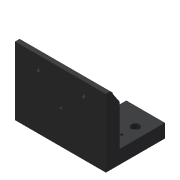
# Autodesk Inventor part: bracket
Saved by Autodesk Inventor 2022 Beta2 (Build 260130000, 130) ContinuousBuild 0
## iProperties
Created: 2006-01-27
Part Number: bracket
Document SubType Name: Modeling
Designer: Dominic
Density: 1 g/cm^3
Material: Generic
Appearance: Generic
Author: dchu
Autodesk Inventor part; units mm, degrees
ref_plane "YZ Plane" through (0, 0, 0) normal (1, 0, 0) x (0, 1, 0)
ref_plane "XZ Plane" through (0, 0, 0) normal (0, 1, 0) x (-1, 0, 0)
sketch "Sketch1" plane through (0, 0, 0) normal (1, 0, 0) x (0, 1, 0)
  line L0 (150.2672, 51.8236) -> (150.2672, 81.8236)
  line L1 (150.2672, 51.8236) -> (20.2672, 51.8236)
  line L2 (20.2672, 51.8236) -> (20.2672, 201.8236)
  line L3 (20.2672, 201.8236) -> (30.2672, 201.8236)
  line L4 (30.2672, 201.8236) -> (50.2672, 172.1724)
  line L5 (50.2672, 172.1724) -> (50.2672, 81.8236)
  line L6 (50.2672, 81.8236) -> (150.2672, 81.8236)
  dimension "d1" = 30
  dimension "d2" = 130
  dimension "d3" = 150
  dimension "d4" = 56
  dimension "d5" = 20
  dimension "d6" = 30
  constraints: 14 end point, 3 perpendicular, 2 parallel
  measures "d1" distance of L0.start L0.end
  measures "d2" distance of L0.start L1.end
  measures "d3" distance of L1.end L2.end
  measures "d4" angle of L4 L3
  measures "d5" distance from line of L5 L3.end
  measures "d6" distance between parallel lines of L5 L2
extrude "Extrusion1" add sketch "Sketch1" along normal blind 200
ref_plane "Work Plane1" through (0, 20.2672, 186.8236) normal (0, 0, -1) x (-1, 0, 0)
sketch "Sketch2" plane through (0, 50.2672, 172.1724) normal (0, 0.829, 0.5592) x (1, 0, 0)
  line L0 (200, -35.7658) -> (200, 0) projected
  circle A0 centre (150, -17.6726) radius 4
  circle A1 centre (50, -17.6726) radius 4
  line L1 (-20, -17.6726) -> (260, -17.6726) projected
  dimension "d10" = 8
  dimension "d11" = 50
  dimension "d12" = 100
  constraints: 2 centre point, 2 point on line, 1 equal radius
  measures "d10" diameter of A0
  measures "d11" distance from line of L0 A0.centre
  measures "d12" distance of A1.centre A0.centre
extrude "Extrusion2" cut sketch "Sketch2" against normal up to next
sketch "Sketch3" plane through (0, 50.2672, 81.8236) normal (0, 0, 1) x (1, 0, 0)
  line L0 (200, 0) -> (200, 100) projected
  line L1 (0, 100) -> (200, 100) projected
  line L2 (0, 100) -> (0, 0) projected
  line L3 (85, 100) -> (115, 100)
  line L4 (115, 100) -> (115, 65.4079)
  line L5 (85, 65.4079) -> (85, 100)
  arc A0 (85, 65.4079) -> (115, 65.4079) centre (100, 65.4079) ccw
  dimension "d15" = 30
  dimension "d16" = 100
  constraints: 6 end point, 2 parallel, 2 point on circle, 1 centre point, 1 collinear, 1 horizontal, 1 perpendicular, 1 tangent
  measures "d15" distance of L3.start L3.end
  measures "d16" distance from line of L0 A0.centre
extrude "Extrusion3" cut sketch "Sketch3" against normal up to next
hole "Hole1" at (175, 80.2672, 81.8236) direction (0, 0, -1) diameter 6 depth 85 tip angle 118
hole "Hole2" at (175, 110.2672, 81.8236) direction (0, 0, -1) diameter 9 depth 30 tip angle 118 counterbore diameter 18 counterbore depth 11
hole "Hole3" at (25, 80.2672, 81.8236) direction (0, 0, -1) diameter 9 depth 30 tip angle 118 counterbore diameter 18 counterbore depth 11
hole "Hole4" at (25, 110.2672, 81.8236) direction (0, 0, -1) diameter 6 depth 30 tip angle 118
hole "Hole5" at (100, 50.2672, 127.1724) direction (0, -1, 0) diameter 8 depth 30 tip angle 118 counterbore diameter 20 counterbore depth 11
body "Solid1"
